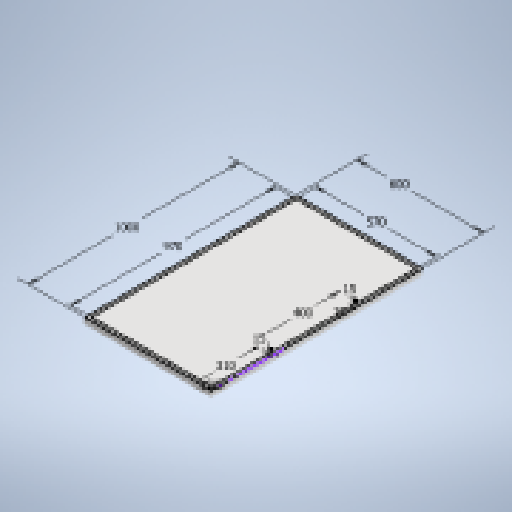
# Autodesk Inventor part: Body Actuator
Saved by Autodesk Inventor 2024 (Build 280153000, 153)
## iProperties
Created: 2024-10-15
Part Number: Body Actuator
Material: 一般
Document SubType Name: Modeling
Designer: jerry
Density: 1 g/cm^3
Appearance: 預設
Author: jerry
Autodesk Inventor part; units mm, degrees
ref_plane "YZ Plane" through (0, 0, 0) normal (1, 0, 0) x (0, 1, 0)
ref_plane "XZ Plane" through (0, 0, 0) normal (0, 1, 0) x (-1, 0, 0)
ref_plane "XY Plane" through (0, 0, 0) normal (0, 0, 1) x (1, 0, 0)
sketch "草圖1" plane through (0, 0, 0) normal (0, 1, 0) x (-1, 0, 0)
  line L0 (0, 0) -> (600, 0)
  line L1 (600, 0) -> (600, -1000)
  line L2 (600, -1000) -> (0, -1000)
  line L3 (0, -1000) -> (0, 0)
  line L4 (0, 0) -> (30, 0)
  line L5 (0, -310) -> (0, 0)
  line L6 (0, -710) -> (0, -310)
  circle A0 centre (30, -310) radius 7.5
  circle A1 centre (30, -710) radius 7.5
  line L7 (0, 0) -> (15, 0)
  line L8 (15, 0) -> (15, -15)
  line L9 (15, -15) -> (0, -15)
  line L10 (0, -15) -> (0, 0)
  line L11 (15, -15) -> (585, -15)
  line L12 (585, -15) -> (585, -985)
  line L13 (585, -985) -> (15, -985)
  line L14 (15, -985) -> (15, -15)
  circle A2 centre (30, -710) radius 3
  circle A3 centre (30, -310) radius 3
  dimension "d0" = 1000
  dimension "d1" = 600
  dimension "d6" = 15
  dimension "d7" = 15
  dimension "d8" = 310
  dimension "d9" = 30
  dimension "d10" = 400
  dimension "d11" = 30
  dimension "d14" = 15
  dimension "d15" = 15
  dimension "d16" = 570
  dimension "d17" = 970
  dimension "d26" = 6
  dimension "d27" = 6
  constraints: 30 end point, 6 parallel, 4 centre point, 4 horizontal, 3 perpendicular, 2 coincident
  measures "d0" distance of L0.end L1.end
  measures "d1" distance of L1.end L2.end
  measures "d6" diameter of A0
  measures "d7" diameter of A1
  measures "d8" distance from line of L0 A0.centre
  measures "d9" distance from line of L3 A0.centre
  measures "d10" distance of A1.centre A0.centre
  measures "d11" distance from line of L3 A1.centre
  measures "d14" distance of L8.end L9.end
  measures "d15" distance of L7.end L8.end
  measures "d16" distance of L12.end L13.end
  measures "d17" distance of L11.end L12.end
  measures "d26" diameter of A2
  measures "d27" diameter of A3
extrude "擠出1" add sketch "草圖1" against normal blind 30 contours L0 L8 L9 L3 | L11 L12 L13 L14 | L0 L1 L2 L3 L9 L8
extrude "擠出2" add sketch "草圖1" against normal blind 30 contours A0 | A1 | A2 | A3
extrude "擠出3" cut sketch "草圖1" against normal blind 25 contours L11 L12 L13 L14
extrude "擠出4" add sketch "草圖1" against normal blind 5 contours L0 L8 L9 L3 | L11 L12 L13 L14 | L0 L1 L2 L3 L9 L8 | A0 | A1 | A2 | A3
extrude "擠出5" cut sketch "草圖1" against normal blind 25 contours A0 | A1 | A2 | A3
extrude "擠出6" cut sketch "草圖1" against normal through all contours A2 | A3
